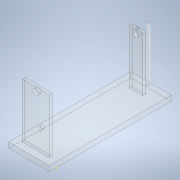
# Autodesk Inventor part: LStand
Saved by Autodesk Inventor 2022 (Build 260153000, 153)
## iProperties
Created: 2023-06-18
Part Number: LStand
Material: PMMA Plastic
Document SubType Name: Modeling
Designer: Preeti Anand
Density: 1.188 g/cm^3
Appearance: Polycarbonate - Clear
Author: Preeti Anand
Autodesk Inventor part; units mm, degrees
ref_plane "YZ Plane" through (0, 0, 0) normal (1, 0, 0) x (0, 1, 0)
ref_plane "XZ Plane" through (0, 0, 0) normal (0, 1, 0) x (-1, 0, 0)
ref_plane "XY Plane" through (0, 0, 0) normal (0, 0, 1) x (1, 0, 0)
sketch "Sketch1" plane through (0, 0, 0) normal (0, 1, 0) x (-1, 0, 0)
  line L0 (0, 0) -> (0, -300)
  line L1 (0, -300) -> (150, -300)
  line L2 (150, -300) -> (150, 0)
  line L3 (150, 0) -> (0, 0)
  dimension "d0" = 300
  dimension "d1" = 150
  dimension "d2" = 300
  dimension "d3" = 150
  constraints: 8 end point, 2 perpendicular, 1 vertical
  measures "d0" distance of L0.start L0.end
  measures "d1" distance of L0.end L1.end
  measures "d2" distance of L1.end L2.end
  measures "d3" distance of L2.end L0.start
extrude "Extrusion1" add sketch "Sketch1" along normal blind 20
sketch "Sketch2" plane through (0, 20, 0) normal (0, 1, 0) x (1, 0, 0)
  line L0 (-25, 35) -> (-125, 35)
  line L1 (-125, 35) -> (-125, 25)
  line L2 (-125, 25) -> (-25, 25)
  line L3 (-25, 25) -> (-25, 35)
  line L4 (-25, 35) -> (-125, 25) construction
  line L5 (-125, 35) -> (-25, 25) construction
  point P0 (0, 0)
  point P1 (-75, 30)
  dimension "d6" = 100
  dimension "d7" = 10
  constraints: 12 end point, 2 midpoint, 2 parallel, 1 horizontal, 1 perpendicular
  measures "d6" distance of L2.end L1.end
  measures "d7" distance of L1.end L0.end
extrude "Extrusion2" add sketch "Sketch2" along normal blind 201.5875
sketch "Sketch3" plane through (-25, 20, -35) normal (0, 0, -1) x (-1, 0, 0)
  circle A0 centre (35, 75) radius 7.5
  point P0 (-25, -20)
  dimension "d10" = 15
  constraints: 1 centre point
  measures "d10" diameter of A0
extrude "Extrusion3" cut sketch "Sketch3" against normal blind 200
sketch "Sketch4" plane through (-25, 20, -35) normal (0, 0, -1) x (-1, 0, 0)
  circle A0 centre (50, 185) radius 8.5
  point P0 (-25, -20)
  dimension "d13" = 17
  constraints: 1 centre point
  measures "d13" diameter of A0
extrude "Extrusion4" cut sketch "Sketch4" against normal blind 15
sketch "Sketch5" plane through (0, 0, -300) normal (0, 0, -1) x (-1, 0, 0)
  line L0 (0, 0) -> (0, 20) projected
  line L1 (0, 20) -> (0, 0)
  line L2 (150, 0) -> (0, 0) projected
  line L3 (0, 0) -> (150, 0)
  line L4 (150, 0) -> (150, 20) projected
  line L5 (150, 0) -> (150, 20)
  line L6 (150, 20) -> (0, 20)
  line L7 (125, 20) -> (25, 20) projected
  constraints: 8 end point, 2 collinear, 1 perpendicular, 1 vertical
extrude "Extrusion5" add sketch "Sketch5" along normal blind 150
sketch "Sketch6" plane through (0, 20, 0) normal (0, 1, 0) x (1, 0, 0)
  line L0 (-100, 395) -> (-50, 395)
  line L1 (-50, 395) -> (-50, 405)
  line L2 (-50, 405) -> (-100, 405)
  line L3 (-100, 405) -> (-100, 395)
  line L4 (-100, 395) -> (-50, 405) construction
  line L5 (-50, 395) -> (-100, 405) construction
  point P0 (0, 0)
  point P1 (-75, 400)
  dimension "d18" = 50
  dimension "d19" = 10
  constraints: 12 end point, 2 midpoint, 2 parallel, 1 horizontal, 1 perpendicular
  measures "d18" distance of L2.end L1.end
  measures "d19" distance of L1.end L0.end
extrude "Extrusion6" add sketch "Sketch6" along normal blind 200
sketch "Sketch7" plane through (-100, 20, -395) normal (0, 0, 1) x (1, 0, 0)
  circle A0 centre (25, 185) radius 8.5 projected
  circle A1 centre (25, 185) radius 8.5
  point P0 (100, -20)
  dimension "d22" = 17
  constraints: 1 centre point, 1 coincident
  measures "d22" diameter of A1
extrude "Extrusion7" cut sketch "Sketch7" against normal blind 200
sketch "Sketch8" plane through (0, 221.5875, 0) normal (0, 1, 0) x (1, 0, 0)
  line L0 (-50, 395) -> (-100, 395) projected
  line L1 (-100, 395) -> (-50, 395)
  line L2 (-100, 405) -> (-50, 405) projected
  circle A0 centre (-75, 400) radius 5
  point P0 (0, 0)
  dimension "d25" = 10
  constraints: 2 end point, 1 centre point, 1 collinear
  measures "d25" diameter of A0
extrude "Extrusion8" add sketch "Sketch8" along normal blind 1
sketch "Sketch9" plane through (-125, 20, -25) normal (0, 0, 1) x (1, 0, 0)
  point P0 (125, -20)
sketch "Sketch10" plane through (-125, 20, -25) normal (0, 0, 1) x (1, 0, 0)
  circle A0 centre (50, 185) radius 8.5 projected
  circle A1 centre (50, 185) radius 10.75
  point P0 (125, -20)
  dimension "d28" = 21.5
  constraints: 1 centre point, 1 coincident
  measures "d28" diameter of A1
extrude "Extrusion9" cut sketch "Sketch10" against normal blind 500 contours A0 | A1
sketch "Sketch11" plane through (0, 20, 0) normal (0, 1, 0) x (1, 0, 0)
  circle A0 centre (-75, 400) radius 5 projected
  line L0 (-150, 450) -> (0, 450) projected
  circle A1 centre (-75, 440) radius 5
  point P0 (0, 0)
  dimension "d31" = 10
  constraints: 1 centre point
  measures "d31" diameter of A1
extrude "Extrusion10" add sketch "Sketch11" along normal blind 200 contours A1
body "Solid1"
